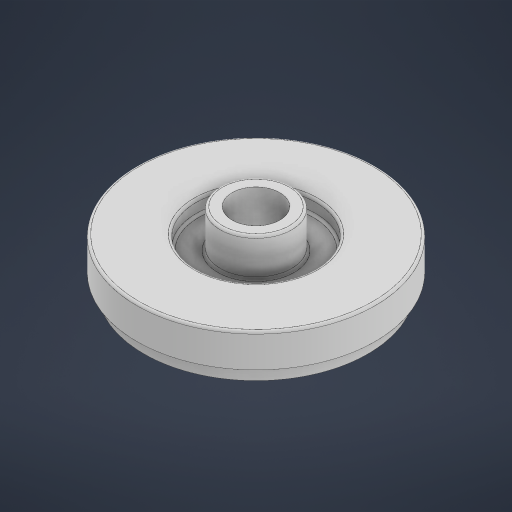
# Autodesk Inventor part: sf_Cylinder_Rear_Lid_1
Saved by Autodesk Inventor 2024 (Build 280153000, 153)
## iProperties
Created: 2024-03-20
Part Number: sf_Cylinder_Rear_Lid_1
Material: Generisch
Document SubType Name: Modeling
Designer: Simon
Density: 1 g/cm^3
Appearance: Vorgabe
Author: Simon
Autodesk Inventor part; units mm, degrees
ref_plane "YZ Plane" through (0, 0, 0) normal (1, 0, 0) x (0, 1, 0)
ref_plane "XZ Plane" through (0, 0, 0) normal (0, 1, 0) x (-1, 0, 0)
ref_plane "XY Plane" through (0, 0, 0) normal (0, 0, 1) x (1, 0, 0)
sketch "Skizze1" plane through (0, 0, 0) normal (1, 0, 0) x (0, 1, 0)
  line L0 (25, -0.5) -> (25, -7)
  line L1 (25, -7) -> (23.5, -7)
  line L2 (23.5, -7) -> (23.5, -10)
  line L3 (23.5, -10) -> (14, -10)
  line L4 (14, -10) -> (14, -13)
  line L5 (14, -13) -> (3, -13)
  line L6 (24.5, 0) -> (13, 0)
  line L7 (12, -3) -> (8, -3)
  line L8 (7.5, -2.5) -> (7.5, 4.5)
  line L9 (7, 5) -> (5, 5)
  line L10 (5, 5) -> (5, -8)
  line L11 (5, -8) -> (3, -8)
  line L12 (3, -13) -> (3, -8)
  arc A0 (12, -3) -> (12.5, -2.5) centre (12, -2.5) ccw
  line L13 (12.5, -0.5) -> (12.5, -2.5)
  arc A1 (13, 0) -> (12.5, -0.5) centre (13, -0.5) ccw
  arc A2 (7.5, -2.5) -> (8, -3) centre (8, -2.5) ccw
  arc A3 (7.5, 4.5) -> (7, 5) centre (7, 4.5) ccw
  arc A4 (25, -0.5) -> (24.5, 0) centre (24.5, -0.5) ccw
  line L14 (0, 0) -> (0, -2.0736) construction
  point P0 (25, 0)
  point P1 (12.5, 0)
  point P2 (7.5, -3)
  point P3 (7.5, 5)
  dimension "d5" = 7
  dimension "d6" = 3
  dimension "d7" = 3
  dimension "d11" = 8
  dimension "d12" = 13
  dimension "d13" = 5
  dimension "d14" = 11
  dimension "d15" = 12.5
  dimension "d16" = 9.5
  dimension "d18" = 0.5
  dimension "d19" = 0.5
  constraints: 30 end point, 12 perpendicular, 10 point on circle, 9 tangent, 8 point on line, 5 centre point, 3 equal radius, 2 vertical
  measures "d5" distance of point (25, 0) L0.end
  measures "d6" distance of L1.end L2.end
  measures "d7" distance of L3.end L4.end
  measures "d11" distance of point (7.5, -3) point (7.5, 5)
  measures "d12" distance of L9.end L10.end
  measures "d13" distance of L5.end L11.end
  measures "d14" distance of L4.end L5.end
  measures "d15" distance of point (25, 0) point (12.5, 0)
  measures "d16" distance of L2.end L3.end
  measures "d18" radius of A0
  measures "d19" radius of A1
revolve "Umdrehung1" add sketch "Skizze1" angle 360 about axis through (0, 0, 0) along (0, 0, -1)
sketch "Skizze2" plane through (0, 0, -8) normal (0, 0, 1) x (1, 0, 0)
  circle A0 centre (0, 0) radius 3 projected
  circle A1 centre (0, 0) radius 5 projected
extrude "Extrusion1" add sketch "Skizze2" along normal blind 4 separate body
